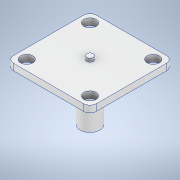
# Autodesk Inventor part: connector
Saved by Autodesk Inventor 2022 (Build 260153000, 153)
## iProperties
Created: 2022-04-25
Part Number: connector
Material: Aluminum 6061
Document SubType Name: Modeling
Designer: Bowen
Density: 2.7 g/cm^3
Appearance: Aluminum - Flat
Author: Bowen
Autodesk Inventor part; units mm, degrees
ref_plane "YZ Plane" through (0, 0, 0) normal (1, 0, 0) x (0, 1, 0)
ref_plane "XZ Plane" through (0, 0, 0) normal (0, 1, 0) x (-1, 0, 0)
ref_plane "XY Plane" through (0, 0, 0) normal (0, 0, 1) x (1, 0, 0)
sketch "Sketch1" plane through (0, 0, 0) normal (0, 1, 0) x (-1, 0, 0)
  line L0 (12.55, 12.55) -> (-12.55, 12.55)
  line L1 (-12.55, 12.55) -> (-12.55, -12.55)
  line L2 (-12.55, -12.55) -> (12.55, -12.55)
  line L3 (12.55, -12.55) -> (12.55, 12.55)
  point P0 (0, 0)
  point P1 (12.55, 0)
  point P2 (0, -12.55)
  dimension "d0" = 25.1
  dimension "d1" = 25.1
  constraints: 8 end point, 2 midpoint, 2 parallel, 1 horizontal, 1 horizontal alignment, 1 perpendicular, 1 vertical alignment
  measures "d0" distance of L2.end L1.end
  measures "d1" distance of L1.end L0.end
extrude "Extrusion1" add sketch "Sketch1" along normal blind 2
fillet "Fillet1" radius 2 4 edges at (12.55, 1, 12.55) (-12.55, 1, 12.55) (12.55, 1, -12.55) (-12.55, 1, -12.55)
sketch "Sketch2" plane through (0, 2, 0) normal (0, 1, 0) x (1, 0, 0)
  circle A0 centre (-9.55, -9.55) radius 1.85
  line L0 (-12.55, 10.55) -> (-12.55, -10.55) projected
  line L1 (-10.55, -12.55) -> (10.55, -12.55) projected
  line L2 (0, 0) -> (-4.3818, 0) construction
  line L3 (0, 0) -> (0, 4.1079) construction
  circle A1 centre (-9.55, 9.55) radius 1.85
  circle A2 centre (9.55, -9.55) radius 1.85
  circle A3 centre (9.55, 9.55) radius 1.85
  dimension "d5" = 3.7
  dimension "d6" = 3
  dimension "d7" = 3
  constraints: 4 centre point, 4 end point, 3 symmetric about line, 1 horizontal, 1 vertical, 3 other
  measures "d5" diameter of A0
  measures "d6" distance from line of L0 A0.centre
  measures "d7" distance from line of L1 A0.centre
extrude "Extrusion2" cut sketch "Sketch2" against normal through all
sketch "Sketch3" plane through (0, 2, 0) normal (0, 1, 0) x (1, 0, 0)
  circle A0 centre (0, 0) radius 1
  dimension "d10" = 2
  constraints: 1 centre point, 1 coincident
  measures "d10" diameter of A0
extrude "Extrusion3" add sketch "Sketch3" along normal blind 1
sketch "Sketch4" plane through (0, 0, 0) normal (0, -1, 0) x (1, 0, 0)
  circle A0 centre (0, 0) radius 1 projected
  circle A1 centre (0, 0) radius 7
  dimension "d13" = 14
  constraints: 1 centre point, 1 coincident
  measures "d13" diameter of A1
extrude "Extrusion4" add sketch "Sketch4" along normal blind 5 contours A0 | A1
sketch "Sketch5" plane through (0, -5, 0) normal (0, -1, 0) x (1, 0, 0)
  circle A0 centre (0, 0) radius 1 projected
  circle A1 centre (0, 0) radius 3
  dimension "d16" = 6
  constraints: 1 centre point, 1 coincident
  measures "d16" diameter of A1
extrude "Extrusion5" add sketch "Sketch5" along normal blind 10 contours A0 | A1
body "Solid1"
